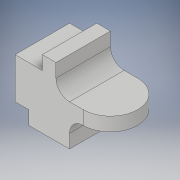
# Autodesk Inventor part: 零件21
Saved by Autodesk Inventor 2019 (Build 230136000, 136)
## iProperties
Created: 2020-09-18
Part Number: 零件21
Material: 一般
Document SubType Name: Modeling
Designer: jay
Density: 1 g/cm^3
Appearance: 預設
Author: jay
Autodesk Inventor part; units mm, degrees
ref_plane "YZ Plane" through (0, 0, 0) normal (1, 0, 0) x (0, 1, 0)
ref_plane "XZ Plane" through (0, 0, 0) normal (0, 1, 0) x (-1, 0, 0)
ref_plane "XY Plane" through (0, 0, 0) normal (0, 0, 1) x (1, 0, 0)
sketch "草圖1" plane through (0, 0, 0) normal (0, 0, 1) x (1, 0, 0)
  line L0 (-14, 0) -> (84, 0) projected
  line L1 (0, -10) -> (0, 60) projected
  line L2 (0, 10) -> (0, 40)
  line L3 (0, 40) -> (20, 40)
  line L4 (20, 40) -> (20, 50)
  line L5 (20, 50) -> (30, 50)
  line L6 (30, 50) -> (30, 30)
  line L7 (30, 30) -> (70, 30)
  line L8 (70, 30) -> (70, 20)
  line L9 (70, 20) -> (40, 20)
  line L10 (40, 20) -> (40, 0)
  line L11 (40, 0) -> (10, 0)
  line L12 (10, 0) -> (10, 10)
  line L13 (10, 10) -> (0, 10)
  point P0 (0, 0)
  dimension "d0" = 50
  dimension "d1" = 10
  dimension "d2" = 20
  dimension "d3" = 70
  dimension "d4" = 30
  dimension "d5" = 10
  dimension "d6" = 10
  dimension "d7" = 30
  dimension "d8" = 20
  dimension "d9" = 40
  constraints: 24 end point, 8 perpendicular, 4 point on line, 1 horizontal, 1 vertical
  measures "d0" distance between parallel lines of L0 L5
  measures "d1" distance of L7.end L8.end
  measures "d2" distance of L9.end L10.end
  measures "d3" distance between parallel lines of L2 L8
  measures "d4" distance of L10.end L11.end
  measures "d5" distance of L11.end L12.end
  measures "d6" distance of L12.end L2.start
  measures "d7" distance of L2.start L2.end
  measures "d8" distance of L2.end L3.end
  measures "d9" distance of L6.end L7.end
extrude "擠出1" add sketch "草圖1" along normal mid plane 40 contours L12 L13 L1 L3 L4 L5 L6 L7 L8 L9 L10 L0
fillet "圓角1" radius 20 2 edges at (70, 25, 20) (70, 25, -20)
fillet "圓角2" radius 10 1 edges at (40, 20, 0)
fillet "圓角3" radius 10 1 edges at (30, 30, 0)
